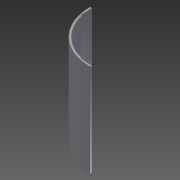
# Autodesk Inventor part: skin.25
Saved by Autodesk Inventor 2011 (Build 150239000, 239)
## iProperties
Created: 2011-01-27
Part Number: skin.25
Document SubType Name: Modeling
Designer: Physics Student
Density: 1 g/cm^3
Author: Physics Student
Autodesk Inventor part; units mm, degrees
ref_plane "YZ Plane" through (0, 0, 0) normal (1, 0, 0) x (0, 1, 0)
ref_plane "XZ Plane" through (0, 0, 0) normal (0, 1, 0) x (-1, 0, 0)
ref_plane "XY Plane" through (0, 0, 0) normal (0, 0, 1) x (1, 0, 0)
sketch "Sketch1" plane through (0, 0, 0) normal (0, 0, 1) x (1, 0, 0)
  circle A0 centre (0, 0) radius 177.8
  circle A1 centre (0, 0) radius 171.45
  dimension "d0" = 355.6
  dimension "d1" = 342.9
  constraints: 2 centre point, 2 coincident
  measures "d0" diameter of A0
  measures "d1" diameter of A1
extrude "Extrusion1" add sketch "Sketch1" along normal blind 317.5
sketch "Sketch2" plane through (0, 0, 317.5) normal (0, 0, 1) x (1, 0, 0)
  circle A0 centre (0, 0) radius 171.45 projected
  circle A1 centre (0, 0) radius 177.8 projected
  line L0 (0, 0) -> (-195.3507, 0)
  line L1 (-170.18, -40) -> (-165.608, -40)
  line L2 (-165.608, -40) -> (-165.608, 40)
  line L3 (-165.608, 40) -> (-170.18, 40)
  line L4 (-170.18, 40) -> (-170.18, -40)
  dimension "d4" = 80
  dimension "d5" = 165.608
  dimension "d6" = 4.572
  constraints: 10 end point, 2 horizontal, 2 parallel, 1 perpendicular, 1 other
  measures "d4" distance of L2.end L1.end
  measures "d5" distance from line of A0.centre L2
  measures "d6" distance between parallel lines of L2 L4
extrude "Extrusion2" cut sketch "Sketch2" against normal blind 317.5 contours L3 L2 L0 L4 A0 | A0 L4 L3 | L1 L4 A0 | A0 L4 L0 L2 L1
pattern_circular "Circular Pattern1" count 4 over 360 about axis through (0, 0, -10) along (0, 0, 1) of "Extrusion2"
sketch "Sketch3" plane through (0, 0, 317.5) normal (0, 0, 1) x (1, 0, 0)
  line L0 (-205.5346, 0) -> (309.1067, 0)
  line L1 (309.1067, 0) -> (309.1067, 465.2654)
  line L2 (309.1067, 465.2654) -> (-205.5346, 465.2654)
  line L3 (-205.5346, 465.2654) -> (-205.5346, 0)
  line L4 (0, 604.1533) -> (225.7004, 604.1533)
  line L5 (225.7004, 604.1533) -> (225.7004, -403.3158)
  line L6 (225.7004, -403.3158) -> (0, -403.3158)
  line L7 (0, -403.3158) -> (0, 604.1533)
  constraints: 16 end point, 4 parallel, 2 horizontal, 2 perpendicular
extrude "Extrusion3" cut sketch "Sketch3" against normal blind 317.5
body "Solid1"
